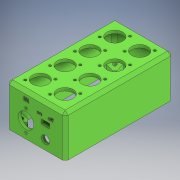
# Autodesk Inventor part: Case1
Saved by Autodesk Inventor 2020 (Build 240168000, 168)
## iProperties
Created: 2020-11-28
Part Number: Case1
Material: Generic
Document SubType Name: Modeling
Designer: Milosz
Density: 1 g/cm^3
Appearance: Default
Author: Milosz
## iProperties of the stored document _3DPrint.ipt
Created: 2020-11-29
Part Number: _3DPrint
Material: Generic
Document SubType Name: Modeling
Designer: Milosz
Density: 1 g/cm^3
Appearance: Default
Author: Milosz
Autodesk Inventor part; units mm, degrees
ref_plane "YZ Plane" through (0, 0, 0) normal (1, 0, 0) x (0, 1, 0)
ref_plane "XZ Plane" through (0, 0, 0) normal (0, 1, 0) x (-1, 0, 0)
ref_plane "XY Plane" through (0, 0, 0) normal (0, 0, 1) x (1, 0, 0)
sketch "Sketch1" plane through (0, 0, 0) normal (0, 1, 0) x (-1, 0, 0)
  circle A0 centre (21.5, -16.9) radius 8
  circle A1 centre (14.2219, -24.8454) radius 1.25
  circle A2 centre (28.7781, -8.9546) radius 1.25
  arc A3 (11.0876, -24.5315) -> (14.8089, -27.9403) centre (14.2219, -24.8454) ccw construction
  arc A4 (31.9108, -9.2842) -> (28.1911, -5.8597) centre (28.7781, -8.9546) ccw construction
  line L0 (31.0995, -16.9941) -> (31.9108, -9.2842) construction
  line L1 (28.1911, -5.8597) -> (19.7111, -7.4682) construction
  line L2 (11.9478, -15.9432) -> (11.0876, -24.5315) construction
  line L3 (23.2889, -26.3318) -> (14.8089, -27.9403) construction
  arc A5 (19.7111, -7.4682) -> (11.9478, -15.9432) centre (21.5, -16.9) ccw construction
  arc A6 (23.2889, -26.3318) -> (31.0995, -16.9941) centre (21.5, -16.9) ccw construction
  line L4 (35.5, -91.9) -> (35.5, -105.9) construction
  line L5 (35.5, -105.9) -> (21.5, -105.9) construction
  line L6 (-3.5, -16.9) -> (-17.5, -16.9) construction
  line L7 (-17.5, -16.9) -> (-17.5, -2.9) construction
  line L8 (-17.5, -2.9) -> (-3.5, -2.9) construction
  line L9 (-3.5, -2.9) -> (-3.5, -16.9) construction
  line L10 (35.5, -105.9) -> (-17.5, -105.9)
  line L11 (-17.5, -105.9) -> (-17.5, -2.9)
  line L12 (-17.5, -2.9) -> (35.5, -2.9)
  line L13 (35.5, -2.9) -> (35.5, -105.9)
  line L14 (28.1911, -30.8597) -> (19.7111, -32.4682) construction
  line L15 (23.2889, -51.3318) -> (14.8089, -52.9403) construction
  circle A7 centre (14.2219, -49.8454) radius 1.25
  circle A8 centre (28.7781, -33.9546) radius 1.25
  line L16 (31.0995, -41.9941) -> (31.9108, -34.2842) construction
  line L17 (11.9478, -40.9432) -> (11.0876, -49.5315) construction
  arc A9 (19.7111, -32.4682) -> (11.9478, -40.9432) centre (21.5, -41.9) ccw construction
  circle A10 centre (21.5, -41.9) radius 8
  arc A11 (11.0876, -49.5315) -> (14.8089, -52.9403) centre (14.2219, -49.8454) ccw construction
  arc A12 (31.9108, -34.2842) -> (28.1911, -30.8597) centre (28.7781, -33.9546) ccw construction
  arc A13 (23.2889, -51.3318) -> (31.0995, -41.9941) centre (21.5, -41.9) ccw construction
  line L18 (28.1911, -55.8597) -> (19.7111, -57.4682) construction
  line L19 (23.2889, -76.3318) -> (14.8089, -77.9403) construction
  circle A14 centre (14.2219, -74.8454) radius 1.25
  circle A15 centre (28.7781, -58.9546) radius 1.25
  line L20 (31.0995, -66.9941) -> (31.9108, -59.2842) construction
  line L21 (11.9478, -65.9432) -> (11.0876, -74.5315) construction
  arc A16 (19.7111, -57.4682) -> (11.9478, -65.9432) centre (21.5, -66.9) ccw construction
  circle A17 centre (21.5, -66.9) radius 8
  arc A18 (11.0876, -74.5315) -> (14.8089, -77.9403) centre (14.2219, -74.8454) ccw construction
  arc A19 (31.9108, -59.2842) -> (28.1911, -55.8597) centre (28.7781, -58.9546) ccw construction
  arc A20 (23.2889, -76.3318) -> (31.0995, -66.9941) centre (21.5, -66.9) ccw construction
  line L22 (28.1911, -80.8597) -> (19.7111, -82.4682) construction
  line L23 (23.2889, -101.3318) -> (14.8089, -102.9403) construction
  circle A21 centre (14.2219, -99.8454) radius 1.25
  circle A22 centre (28.7781, -83.9546) radius 1.25
  line L24 (31.0995, -91.9941) -> (31.9108, -84.2842) construction
  line L25 (11.9478, -90.9432) -> (11.0876, -99.5315) construction
  arc A23 (19.7111, -82.4682) -> (11.9478, -90.9432) centre (21.5, -91.9) ccw construction
  circle A24 centre (21.5, -91.9) radius 8
  arc A25 (11.0876, -99.5315) -> (14.8089, -102.9403) centre (14.2219, -99.8454) ccw construction
  arc A26 (31.9108, -84.2842) -> (28.1911, -80.8597) centre (28.7781, -83.9546) ccw construction
  arc A27 (23.2889, -101.3318) -> (31.0995, -91.9941) centre (21.5, -91.9) ccw construction
  line L26 (3.1911, -5.8597) -> (-5.2889, -7.4682) construction
  line L27 (-1.7111, -26.3318) -> (-10.1911, -27.9403) construction
  circle A28 centre (-10.7781, -24.8454) radius 1.25
  circle A29 centre (3.7781, -8.9546) radius 1.25
  line L28 (6.0995, -16.9941) -> (6.9108, -9.2842) construction
  line L29 (-13.0522, -15.9432) -> (-13.9124, -24.5315) construction
  arc A30 (-5.2889, -7.4682) -> (-13.0522, -15.9432) centre (-3.5, -16.9) ccw construction
  circle A31 centre (-3.5, -16.9) radius 8
  arc A32 (-13.9124, -24.5315) -> (-10.1911, -27.9403) centre (-10.7781, -24.8454) ccw construction
  arc A33 (6.9108, -9.2842) -> (3.1911, -5.8597) centre (3.7781, -8.9546) ccw construction
  arc A34 (-1.7111, -26.3318) -> (6.0995, -16.9941) centre (-3.5, -16.9) ccw construction
  line L30 (3.1911, -30.8597) -> (-5.2889, -32.4682) construction
  line L31 (-1.7111, -51.3318) -> (-10.1911, -52.9403) construction
  circle A35 centre (-10.7781, -49.8454) radius 1.25
  circle A36 centre (3.7781, -33.9546) radius 1.25
  line L32 (6.0995, -41.9941) -> (6.9108, -34.2842) construction
  line L33 (-13.0522, -40.9432) -> (-13.9124, -49.5315) construction
  arc A37 (-5.2889, -32.4682) -> (-13.0522, -40.9432) centre (-3.5, -41.9) ccw construction
  circle A38 centre (-3.5, -41.9) radius 8
  arc A39 (-13.9124, -49.5315) -> (-10.1911, -52.9403) centre (-10.7781, -49.8454) ccw construction
  arc A40 (6.9108, -34.2842) -> (3.1911, -30.8597) centre (3.7781, -33.9546) ccw construction
  arc A41 (-1.7111, -51.3318) -> (6.0995, -41.9941) centre (-3.5, -41.9) ccw construction
  line L34 (3.1911, -55.8597) -> (-5.2889, -57.4682) construction
  line L35 (-1.7111, -76.3318) -> (-10.1911, -77.9403) construction
  circle A42 centre (-10.7781, -74.8454) radius 1.25
  circle A43 centre (3.7781, -58.9546) radius 1.25
  line L36 (6.0995, -66.9941) -> (6.9108, -59.2842) construction
  line L37 (-13.0522, -65.9432) -> (-13.9124, -74.5315) construction
  arc A44 (-5.2889, -57.4682) -> (-13.0522, -65.9432) centre (-3.5, -66.9) ccw construction
  circle A45 centre (-3.5, -66.9) radius 8
  arc A46 (-13.9124, -74.5315) -> (-10.1911, -77.9403) centre (-10.7781, -74.8454) ccw construction
  arc A47 (6.9108, -59.2842) -> (3.1911, -55.8597) centre (3.7781, -58.9546) ccw construction
  arc A48 (-1.7111, -76.3318) -> (6.0995, -66.9941) centre (-3.5, -66.9) ccw construction
  line L38 (3.1911, -80.8597) -> (-5.2889, -82.4682) construction
  line L39 (-1.7111, -101.3318) -> (-10.1911, -102.9403) construction
  circle A49 centre (-10.7781, -99.8454) radius 1.25
  circle A50 centre (3.7781, -83.9546) radius 1.25
  line L40 (6.0995, -91.9941) -> (6.9108, -84.2842) construction
  line L41 (-13.0522, -90.9432) -> (-13.9124, -99.5315) construction
  arc A51 (-5.2889, -82.4682) -> (-13.0522, -90.9432) centre (-3.5, -91.9) ccw construction
  circle A52 centre (-3.5, -91.9) radius 8
  arc A53 (-13.9124, -99.5315) -> (-10.1911, -102.9403) centre (-10.7781, -99.8454) ccw construction
  arc A54 (6.9108, -84.2842) -> (3.1911, -80.8597) centre (3.7781, -83.9546) ccw construction
  arc A55 (-1.7111, -101.3318) -> (6.0995, -91.9941) centre (-3.5, -91.9) ccw construction
  line L42 (28.7781, -8.9546) -> (14.2219, -24.8454) construction
  point P0 (0, 0)
  point P1 (21.5, -16.9)
  point P2 (21.5, -41.9)
  point P3 (21.5, -66.9)
  point P4 (21.5, -91.9)
  point P5 (-3.5, -41.9)
  point P6 (-3.5, -66.9)
  point P7 (-3.5, -91.9)
  dimension "d0" = 16
  dimension "d3" = 2.5
  dimension "d4" = 2.5
  dimension "d6" = 6.3
  dimension "d7" = 6.3
  dimension "d9" = 9.6
  dimension "d10" = 9.6
  dimension "d19" = 14
  dimension "d20" = 14
  dimension "d21" = 14
  dimension "d22" = 14
  dimension "d25" = 25
  dimension "d28" = 25
  dimension "d55" = 10.775
  dimension "d56" = 10.775
  constraints: 86 end point, 64 point on circle, 56 centre point, 24 coincident, 7 tangent, 4 parallel, 3 horizontal, 2 perpendicular, 1 midpoint, 1 vertical, 182 other
  measures "d0" diameter of A0
  measures "d3" diameter of A1
  measures "d4" diameter of A2
  measures "d6" diameter of A3
  measures "d7" diameter of A4
  measures "d9" radius of A6
  measures "d10" radius of A5
  measures "d19" distance of L4.end L5.end
  measures "d20" distance of L4.start L4.end
  measures "d21" distance of L7.end L8.end
  measures "d22" distance of L6.end L7.end
  measures "d25" distance of L2.start L17.start
  measures "d28" distance of L2.start L29.start
  measures "d55" distance of A0.centre A1.centre
  measures "d56" distance of A2.centre A0.centre
extrude "Extrusion1" add sketch "Sketch1" along normal blind 3
sketch "Sketch2" plane through (0, 0, 0) normal (0, -1, 0) x (1, 0, 0)
  line L0 (-35.5, -105.9) -> (-35.5, -2.9) projected
  line L1 (-35.5, -2.9) -> (17.5, -2.9) projected
  line L2 (-35.5, -2.9) -> (17.5, -2.9) projected
  line L3 (17.5, -2.9) -> (-35.5, -2.9)
  line L4 (-35.5, -2.9) -> (-35.5, 0.1)
  line L5 (-35.5, 0.1) -> (17.5, 0.1)
  line L6 (17.5, 0.1) -> (17.5, -2.9)
  line L7 (-35.5, 0.1) -> (-38.5, 0.1)
  line L8 (-38.5, 0.1) -> (-38.5, -105.9)
  line L9 (-38.5, -105.9) -> (-35.5, -105.9)
  line L10 (-35.5, -105.9) -> (-35.5, 0.1)
  line L11 (-38.5, -105.9) -> (17.5, -105.9)
  line L12 (17.5, -105.9) -> (17.5, -108.9)
  line L13 (17.5, -108.9) -> (-38.5, -108.9)
  line L14 (-38.5, -108.9) -> (-38.5, -105.9)
  line L15 (17.5, -108.9) -> (20.5, -108.9)
  line L16 (20.5, -108.9) -> (20.5, 0.1)
  line L17 (20.5, 0.1) -> (17.5, 0.1)
  line L18 (17.5, 0.1) -> (17.5, -108.9)
  point P0 (0, 0)
  point P1 (17.5, -2.9)
  dimension "d33" = 3
  dimension "d34" = 3
  dimension "d35" = 3
  dimension "d36" = 3
  constraints: 32 end point, 8 parallel, 4 horizontal, 4 perpendicular, 2 point on line
  measures "d33" distance of L3.end L4.end
  measures "d34" distance of L9.end L8.end
  measures "d35" distance of L11.end L12.end
  measures "d36" distance of L17.end L16.end
extrude "Extrusion2" add sketch "Sketch2" along normal blind 40 and the other way blind 3 contours L9 L8 L7 L4 L0 | L11 L12 L13 L14 L9 | L4 L5 L6 L1 | L18 L6 L17 L16 L15 L12
chamfer "Chamfer1" distance 3 angle 45 16 edges at (-9, 3, 0.1) (-38.5, 3, -54.4) (-9, 3, -108.9) (20.5, 3, -54.4) (20.5, -18.5, -108.9) (-38.5, -18.5, -108.9) (20.5, -18.5, 0.1) (-38.5, -18.5, 0.1) (-35.5, -20, -2.9) (17.5, -20, -2.9) (17.5, -20, -105.9) (-35.5, -20, -105.9) (-9, 0, -2.9) (-35.5, 0, -54.4) (-9, 0, -105.9) (17.5, 0, -54.4)
sketch "Sketch3" plane through (0, 0, 0) normal (0, -1, 0) x (1, 0, 0)
  circle A0 centre (3.5, -91.9) radius 8 projected
  circle A1 centre (-3.7781, -83.9546) radius 1.25 projected
  circle A2 centre (10.7781, -99.8454) radius 1.25 projected
  circle A3 centre (3.5, -66.9) radius 8 projected
  circle A4 centre (-3.7781, -58.9546) radius 1.25 projected
  circle A5 centre (10.7781, -74.8454) radius 1.25 projected
  circle A6 centre (3.5, -41.9) radius 8 projected
  circle A7 centre (-3.7781, -33.9546) radius 1.25 projected
  circle A8 centre (10.7781, -49.8454) radius 1.25 projected
  circle A9 centre (3.5, -16.9) radius 8 projected
  circle A10 centre (-3.7781, -8.9546) radius 1.25 projected
  circle A11 centre (10.7781, -24.8454) radius 1.25 projected
  circle A12 centre (-21.5, -91.9) radius 8 projected
  circle A13 centre (-28.7781, -83.9546) radius 1.25 projected
  circle A14 centre (-14.2219, -99.8454) radius 1.25 projected
  circle A15 centre (-21.5, -66.9) radius 8 projected
  circle A16 centre (-28.7781, -58.9546) radius 1.25 projected
  circle A17 centre (-14.2219, -74.8454) radius 1.25 projected
  circle A18 centre (-21.5, -41.9) radius 8 projected
  circle A19 centre (-28.7781, -33.9546) radius 1.25 projected
  circle A20 centre (-14.2219, -49.8454) radius 1.25 projected
  circle A21 centre (-28.7781, -8.9546) radius 1.25 projected
  circle A22 centre (-14.2219, -24.8454) radius 1.25 projected
  circle A23 centre (-21.5, -16.9) radius 8 projected
  line L0 (14.5, -102.9) -> (-32.5, -102.9) projected
  line L1 (14.5, -5.9) -> (14.5, -102.9) projected
  line L2 (-32.5, -5.9) -> (14.5, -5.9) projected
  line L3 (-32.5, -102.9) -> (-32.5, -5.9) projected
  line L4 (-14.2219, -24.8454) -> (-21.5, -16.9) construction
  line L5 (-14.7713, -22.3652) -> (-12.3487, -23.1295)
  line L6 (-12.3487, -23.1295) -> (-11.7993, -25.6098)
  line L7 (-11.7993, -25.6098) -> (-13.6725, -27.3257)
  line L8 (-13.6725, -27.3257) -> (-16.0951, -26.5613)
  line L9 (-16.0951, -26.5613) -> (-16.6445, -24.0811)
  line L10 (-16.6445, -24.0811) -> (-14.7713, -22.3652)
  circle A24 centre (-28.7781, -8.9546) radius 1.25 construction
  line L11 (-28.7781, -8.9546) -> (-21.5, -16.9) construction
  line L12 (-28.2287, -11.4348) -> (-30.6513, -10.6705)
  line L13 (-30.6513, -10.6705) -> (-31.2007, -8.1902)
  line L14 (-31.2007, -8.1902) -> (-29.3275, -6.4743)
  line L15 (-29.3275, -6.4743) -> (-26.9049, -7.2387)
  line L16 (-26.9049, -7.2387) -> (-26.3555, -9.7189)
  line L17 (-26.3555, -9.7189) -> (-28.2287, -11.4348)
  point P0 (0, 0)
  point P1 (-14.1712, -24.9007)
  point P2 (-15.7079, -23.2232)
  point P3 (-27.2921, -10.5768)
  dimension "d45" = 4.4
  dimension "d46" = 4.4
  constraints: 28 end point, 2 coincident, 2 midpoint, 2 point on line, 26 other
  measures "d45" distance between parallel lines of L7 L10
  measures "d46" distance between parallel lines of L16 L13
extrude "Extrusion3" cut sketch "Sketch3" against normal blind 1 contours L5 L6 L7 L8 L9 L10 | L12 L13 L14 L15 L16 L17
pattern_linear "Rectangular Pattern1" count 4 spacing 25 along (0, 0, -1) count 2 spacing 25 along (1, 0, 0) of "Extrusion3"
sketch "Sketch4" plane through (0, -40, 0) normal (0, -1, 0) x (1, 0, 0)
  line L0 (17.5, -5.9) -> (17.5, -102.9) projected
  line L1 (17.5, -5.9) -> (17.5, -102.9) projected
  line L2 (14.5, -105.9) -> (17.5, -102.9) projected
  line L3 (14.5, -105.9) -> (-32.5, -105.9) projected
  line L4 (-35.5, -102.9) -> (-32.5, -105.9) projected
  line L5 (-35.5, -102.9) -> (-35.5, -5.9) projected
  line L6 (-32.5, -2.9) -> (-35.5, -5.9) projected
  line L7 (-32.5, -2.9) -> (14.5, -2.9) projected
  line L8 (17.5, -5.9) -> (14.5, -2.9) projected
  line L9 (20.5, -105.9) -> (17.5, -108.9) projected
  line L10 (20.5, -105.9) -> (20.5, -2.9) projected
  line L11 (17.5, 0.1) -> (20.5, -2.9) projected
  line L12 (17.5, 0.1) -> (-35.5, 0.1) projected
  line L13 (-38.5, -2.9) -> (-35.5, 0.1) projected
  line L14 (-38.5, -2.9) -> (-38.5, -105.9) projected
  line L15 (-35.5, -108.9) -> (-38.5, -105.9) projected
  line L16 (-35.5, -108.9) -> (17.5, -108.9) projected
  circle A0 centre (-31.1, -7.3) radius 1.75
  line L17 (-35.5, -2.9) -> (-35.5, -105.9) projected
  line L18 (-35.5, -2.9) -> (-26.7, -2.9)
  line L19 (-26.7, -2.9) -> (-26.7, -11.7)
  line L20 (-26.7, -11.7) -> (-35.5, -11.7)
  line L21 (-35.5, -11.7) -> (-35.5, -2.9)
  point P0 (0, 0)
  dimension "d57" = 3.5
  dimension "d58" = 8.8
  dimension "d59" = 8.8
  dimension "d60" = 4.4
  dimension "d61" = 4.4
  constraints: 8 end point, 2 parallel, 1 centre point, 1 horizontal, 1 perpendicular
  measures "d57" diameter of A0
  measures "d58" distance of L19.end L20.end
  measures "d59" distance of L18.end L19.end
  measures "d60" distance from line of L7 A0.centre
  measures "d61" distance from line of L21 A0.centre
extrude "Extrusion4" add sketch "Sketch4" against normal blind 7.05 contours L19 L20 L5 L6 L7
chamfer "Chamfer2" distance 2 angle 45 1 edges at (-26.7, -36.475, -11.7)
draft "FaceDraft1" angle 30 pull direction (0.7071068, 0, -0.7071068) faces at (-27.6003, -32.95, -6.4937) fixed edges at (-27.7, -32.95, -10.7)
sketch "Sketch5" plane through (0, -40, 0) normal (0, -1, 0) x (1, 0, 0)
  line L0 (20.5, -105.9) -> (17.5, -108.9) projected
  line L1 (20.5, -105.9) -> (20.5, -2.9) projected
  line L2 (17.5, 0.1) -> (20.5, -2.9) projected
  line L3 (17.5, 0.1) -> (-35.5, 0.1) projected
  line L4 (-38.5, -2.9) -> (-35.5, 0.1) projected
  line L5 (-38.5, -2.9) -> (-38.5, -105.9) projected
  line L6 (-35.5, -108.9) -> (-38.5, -105.9) projected
  line L7 (-35.5, -108.9) -> (17.5, -108.9) projected
  line L8 (-26.7, -9.7) -> (-28.7, -11.7) projected
  line L9 (-26.7, -9.7) -> (-26.7, -2.9) projected
  line L10 (-26.7, -2.9) -> (14.5, -2.9) projected
  line L11 (17.5, -5.9) -> (14.5, -2.9) projected
  line L12 (17.5, -5.9) -> (17.5, -102.9) projected
  line L13 (14.5, -105.9) -> (17.5, -102.9) projected
  line L14 (14.5, -105.9) -> (-32.5, -105.9) projected
  line L15 (-35.5, -102.9) -> (-32.5, -105.9) projected
  line L16 (-35.5, -102.9) -> (-35.5, -11.7) projected
  line L17 (-35.5, -11.7) -> (-28.7, -11.7) projected
  circle A0 centre (-31.1, -7.3) radius 1.75 projected
  line L18 (18.95, -3.542) -> (18.95, -105.258)
  line L19 (18.95, -105.258) -> (16.858, -107.35)
  line L20 (16.858, -107.35) -> (-34.858, -107.35)
  line L21 (-34.858, -107.35) -> (-36.95, -105.258)
  line L22 (-36.95, -105.258) -> (-36.95, -3.542)
  line L23 (-36.95, -3.542) -> (-34.858, -1.45)
  line L24 (-34.858, -1.45) -> (16.858, -1.45)
  line L25 (16.858, -1.45) -> (18.95, -3.542)
  point P0 (0, 0)
  dimension "d68" = 1.55
  constraints: 16 end point, 7 other
  measures "d68" distance between parallel lines of L1 L18
extrude "Extrusion5" cut sketch "Sketch5" against normal blind 1 contours L0 L7 L6 L5 L4 L3 L2 L1
sketch "Sketch7" plane through (-26.7, -40, -9.7) normal (0.7071068, 0, -0.7071068) x (-0.7071068, 0, -0.7071068)
  circle A0 centre (1.4142, 13.6083) radius 1.75
  line L0 (3.1642, 0) -> (-0.3358, 0)
  line L1 (3.1642, 0) -> (-0.3358, 13.6083) construction
  circle A1 centre (1.4142, 13.6083) radius 1.75 construction
  line L2 (3.1642, 13.6083) -> (-0.3358, 0) construction
  line L3 (1.4142, 6.8042) -> (1.4142, 0) construction
  line L4 (3.1642, 0) -> (-0.3358, 0) construction
  line L5 (-1.5858, 5.2) -> (4.4142, 5.2)
  line L6 (4.4142, 5.2) -> (4.4142, 2.5)
  line L7 (4.4142, 2.5) -> (-1.5858, 2.5)
  line L8 (-1.5858, 2.5) -> (-1.5858, 5.2)
  line L9 (-1.5858, 5.2) -> (4.4142, 2.5) construction
  line L10 (4.4142, 5.2) -> (-1.5858, 2.5) construction
  line L11 (-0.0651, 0) -> (2.8935, 0) construction
  point P0 (-25.7387, 40)
  point P1 (1.4142, 3.4021)
  point P2 (1.4142, 3.85)
  dimension "d73" = 6
  dimension "d74" = 2.7
  dimension "d75" = 2.5
  constraints: 20 end point, 5 midpoint, 2 parallel, 2 point on circle, 1 centre point, 1 horizontal, 1 perpendicular, 1 point on line, 1 vertical
  measures "d73" distance of L6.end L7.end
  measures "d74" distance of L5.end L6.end
  measures "d75" distance between parallel lines of L11 L7
extrude "Extrusion6" cut sketch "Sketch7" against normal up to surface (8.9095 mm away) contours L5 L6 L7 L8
chamfer "Chamfer3" distance 1 distance2 3 1 edges at (-29.2893, -37.5, -4.868) measured on face at (-29.2893, -37, -4.868)
chamfer "Chamfer4" distance 3 distance2 1 1 edges at (-33.532, -37.5, -9.1107) measured on face at (-33.1784, -37.5, -8.7571)
sketch "Sketch8" plane through (0, -40, 0) normal (0, -1, 0) x (1, 0, 0)
  line L0 (-36.95, -3.542) -> (-36.95, -105.258) projected
  line L1 (-36.95, -105.258) -> (-34.858, -107.35) projected
  line L2 (-34.858, -107.35) -> (16.858, -107.35) projected
  line L3 (16.858, -107.35) -> (18.95, -105.258) projected
  line L4 (18.95, -105.258) -> (18.95, -3.542) projected
  line L5 (18.95, -3.542) -> (16.858, -1.45) projected
  line L6 (16.858, -1.45) -> (-34.858, -1.45) projected
  line L7 (-34.858, -1.45) -> (-36.95, -3.542) projected
  line L8 (-26.7, -9.7) -> (-28.7, -11.7) projected
  line L9 (-26.7, -9.7) -> (-26.7, -2.9) projected
  line L10 (-26.7, -2.9) -> (14.5, -2.9) projected
  line L11 (17.5, -5.9) -> (14.5, -2.9) projected
  line L12 (17.5, -5.9) -> (17.5, -102.9) projected
  line L13 (14.5, -105.9) -> (17.5, -102.9) projected
  line L14 (14.5, -105.9) -> (-32.5, -105.9) projected
  line L15 (-35.5, -102.9) -> (-32.5, -105.9) projected
  line L16 (-35.5, -102.9) -> (-35.5, -11.7) projected
  line L17 (-35.5, -11.7) -> (-28.7, -11.7) projected
  circle A0 centre (-31.1, -7.3) radius 1.75 projected
  line L18 (17.5, -102.9) -> (17.5, -5.9) projected
  line L19 (17.5, -54.4) -> (-35.5, -54.4)
  line L20 (-35.5, -2.9) -> (-35.5, -105.9) projected
  line L21 (14.5, -105.9) -> (-32.5, -105.9) projected
  line L22 (-9, -105.9) -> (-9, -2.9)
  line L23 (-26.7, -2.9) -> (14.5, -2.9) projected
  point P0 (0, 0)
  constraints: 4 end point, 3 midpoint, 1 perpendicular, 1 point on line
ref_plane "Work Plane1" through (17.5, -40, -54.4) normal (0, 0, 1) x (-1, 0, 0)
ref_plane "Work Plane2" through (-9, -40, -105.9) normal (1, 0, 0) x (0, 0, 1)
mirror "Mirror1" about plane through (17.5, -40, -54.4) normal (0, 0, 1) of "Extrusion4", "Chamfer2", "Extrusion6", "Chamfer4", "Chamfer3", "FaceDraft1"
mirror "Mirror2" about plane through (-9, -40, -105.9) normal (1, 0, 0) of "Extrusion6", "Chamfer3", "Chamfer4", "Extrusion4", "FaceDraft1", "Chamfer2", "Mirror1"
sketch "Sketch10" plane through (14.5, -3, -2.9) normal (0, 0, -1) x (-1, 0, 0)
  circle A0 centre (33.25, -19.75) radius 7.75
  line L0 (50, -24.8061) -> (50, 0) projected
  line L1 (47, 3) -> (0, 3) projected
  line L2 (33.25, -5.3373) -> (33.25, -31.7007) construction
  line L3 (-2.358, -37) -> (49.358, -37) construction
  circle A1 centre (33.25, -8.975) radius 1.25
  circle A2 centre (33.25, -30.525) radius 1.25
  line L4 (33.25, -19.75) -> (3.6624, -19.75) construction
  circle A3 centre (13.7076, -26.75) radius 4
  line L5 (13.7076, -26.75) -> (13.7076, -32.2603) construction
  line L6 (13.7076, -26.75) -> (13.7076, -6.8032) construction
  line L7 (9.4576, -10.5) -> (17.9576, -10.5)
  line L8 (17.9576, -10.5) -> (17.9576, -15)
  line L9 (17.9576, -15) -> (9.4576, -15)
  line L10 (9.4576, -15) -> (9.4576, -10.5)
  line L11 (9.4576, -10.5) -> (17.9576, -15) construction
  line L12 (17.9576, -10.5) -> (9.4576, -15) construction
  point P0 (14.5, 3)
  point P1 (13.7076, -12.75)
  dimension "d86" = 15.5
  dimension "d87" = 16.75
  dimension "d88" = 22.75
  dimension "d89" = 2.5
  dimension "d90" = 2.5
  dimension "d91" = 10.775
  dimension "d92" = 10.775
  dimension "d95" = 8
  dimension "d103" = 7
  dimension "d106" = 8.5
  dimension "d107" = 4.5
  dimension "d108" = 7
  constraints: 20 end point, 4 centre point, 3 point on line, 3 vertical, 2 horizontal, 2 midpoint, 2 parallel, 2 perpendicular
  measures "d86" diameter of A0
  measures "d87" distance from line of L0 L4.start
  measures "d88" distance from line of L1 L4.start
  measures "d89" diameter of A1
  measures "d90" diameter of A2
  measures "d91" distance of A2.centre L4.start
  measures "d92" distance of A1.centre L4.start
  measures "d95" diameter of A3
  measures "d103" distance from line of L5.start L4
  measures "d106" distance of L8.end L9.end
  measures "d107" distance of L7.end L8.end
  measures "d108" distance from line of point (13.708, -12.75) L4
extrude "Extrusion7" cut sketch "Sketch10" against normal up to surface (3 mm away) contours A0 | A1 | A2
extrude "Extrusion8" cut sketch "Sketch10" against normal up to surface (3 mm away) contours A3
sketch "Sketch11" plane through (14.5, -3, -2.9) normal (0, 0, -1) x (-1, 0, 0)
  circle A0 centre (13.7076, -26.75) radius 4 projected
  circle A1 centre (33.25, -30.525) radius 1.25 projected
  circle A2 centre (33.25, -19.75) radius 7.75 projected
  circle A3 centre (33.25, -8.975) radius 1.25 projected
  line L0 (50, -36) -> (-3, -36) projected
  line L1 (-3, 3) -> (-3, -36) projected
  line L2 (50, 3) -> (-3, 3) projected
  line L3 (50, -36) -> (50, 3) projected
  circle A4 centre (33.25, -8.975) radius 1.25 construction
  line L4 (33.25, -8.975) -> (33.25, -30.525) construction
  line L5 (31.9798, -11.175) -> (30.7097, -8.975)
  line L6 (30.7097, -8.975) -> (31.9798, -6.775)
  line L7 (31.9798, -6.775) -> (34.5202, -6.775)
  line L8 (34.5202, -6.775) -> (35.7903, -8.975)
  line L9 (35.7903, -8.975) -> (34.5202, -11.175)
  line L10 (34.5202, -11.175) -> (31.9798, -11.175)
  line L11 (34.5202, -28.325) -> (35.7903, -30.525)
  line L12 (35.7903, -30.525) -> (34.5202, -32.725)
  line L13 (34.5202, -32.725) -> (31.9798, -32.725)
  line L14 (31.9798, -32.725) -> (30.7097, -30.525)
  line L15 (30.7097, -30.525) -> (31.9798, -28.325)
  line L16 (31.9798, -28.325) -> (34.5202, -28.325)
  point P0 (14.5, 3)
  point P1 (33.25, -11.175)
  point P2 (33.25, -28.325)
  dimension "d98" = 4.4
  dimension "d99" = 4.4
  constraints: 26 end point, 2 coincident, 2 midpoint, 2 point on line, 1 vertical, 26 other
  measures "d98" distance between parallel lines of L13 L16
  measures "d99" distance between parallel lines of L8 L5
extrude "Extrusion9" cut sketch "Sketch11" against normal blind 1 contours L5 L6 L7 L8 L9 L10 | L11 L12 L13 L14 L15 L16
extrude "Extrusion10" cut sketch "Sketch10" against normal up to surface (3 mm away) contours L7 L8 L9 L10
sketch "Sketch12" plane through (14.5, -3, -2.9) normal (0, 0, -1) x (-1, 0, 0)
  point P0 (14.5, 3)
sketch "Sketch13" plane through (-35.5, 0, 0.1) normal (0, 0, 1) x (1, 0, 0)
  line L0 (13.9336, -2.4788) -> (19.5664, -2.4788) construction
  line L1 (19.5664, -2.4788) -> (19.5664, -8.7517) construction
  line L2 (19.5664, -8.7517) -> (13.9336, -8.7517) construction
  line L3 (13.9336, -8.7517) -> (13.9336, -2.4788) construction
  circle A0 centre (16.75, -22.75) radius 7.75 projected
  line L4 (16.75, -22.75) -> (16.75, -11.7933) construction
  line L5 (13.9336, -2.4788) -> (19.5664, -8.7517) construction
  line L6 (13.9336, -8.7517) -> (19.5664, -2.4788) construction
  line L7 (27.516, -8.5202) -> (33.1488, -8.5202) construction
  line L8 (33.1488, -8.5202) -> (33.1488, -14.7932) construction
  line L9 (33.1488, -14.7932) -> (27.516, -14.7932) construction
  line L10 (27.516, -14.7932) -> (27.516, -8.5202) construction
  line L11 (38.5374, -13.9018) -> (38.5374, -7.6289) construction
  line L12 (38.5374, -7.6289) -> (44.1702, -7.6289) construction
  line L13 (44.1702, -7.6289) -> (44.1702, -13.9018) construction
  line L14 (44.1702, -13.9018) -> (38.5374, -13.9018) construction
  line L15 (40.5424, -18) -> (32.0424, -18) projected
  line L16 (32.0424, -18) -> (32.0424, -13.5) projected
  line L17 (32.0424, -13.5) -> (40.5424, -13.5) projected
  line L18 (40.5424, -13.5) -> (40.5424, -18) projected
  circle A1 centre (36.2924, -29.75) radius 4 projected
  circle A2 centre (16.75, -33.525) radius 1.25 projected
  circle A3 centre (16.75, -22.75) radius 7.75 projected
  circle A4 centre (16.75, -11.975) radius 1.25 projected
  line L19 (0, -39) -> (53, -39) projected
  line L20 (53, 0) -> (53, -39) projected
  line L21 (0, 0) -> (53, 0) projected
  line L22 (0, -39) -> (0, 0) projected
  line L23 (40.5424, -18) -> (32.0424, -13.5) construction
  line L24 (40.5424, -18) -> (32.0424, -18) projected
  line L25 (32.0424, -18) -> (40.5424, -13.5) construction
  line L26 (36.2924, -15.75) -> (36.2924, -7.6059) construction
  spline S0 degree 2 poles (15.1806, -6.3698) (15.1806, -6.3999) (15.1393, -6.4487) (15.0491, -6.4788) (14.8951, -6.4975) (14.775, -6.4975) knots 0 0 0 1 2 3 4 4 4
  spline S1 degree 2 poles (14.775, -6.4975) (14.6585, -6.4975) (14.5008, -6.4788) (14.4106, -6.4487) (14.3693, -6.3999) (14.3693, -6.3698) knots 0 0 0 1 2 3 4 4 4
  line L27 (14.3693, -6.3698) -> (14.3693, -2.6065)
  spline S2 degree 2 poles (14.3693, -2.6065) (14.3693, -2.5764) (14.4106, -2.5276) (14.5045, -2.4975) (14.6585, -2.4788) (14.775, -2.4788) knots 0 0 0 1 2 3 4 4 4
  spline S3 degree 2 poles (14.775, -2.4788) (14.8951, -2.4788) (15.0491, -2.4975) (15.1393, -2.5276) (15.1806, -2.5764) (15.1806, -2.6065) knots 0 0 0 1 2 3 4 4 4
  line L28 (15.1806, -2.6065) -> (15.1806, -6.3698)
  spline S4 degree 2 poles (19.3308, -6.1971) (19.3308, -6.2684) (19.282, -6.3773) (19.1994, -6.4525) (19.0829, -6.4863) (19.0266, -6.4863) knots 0 0 0 1 2 3 4 4 4
  line L29 (19.0266, -6.4863) -> (18.6811, -6.4863)
  spline S5 degree 2 poles (18.6811, -6.4863) (18.5759, -6.4863) (18.4181, -6.4412) (18.2867, -6.3285) (18.1628, -6.1332) (18.0839, -5.983) knots 0 0 0 1 2 3 4 4 4
  line L30 (18.0839, -5.983) -> (17.0923, -4.1201)
  spline S6 degree 2 poles (17.0923, -4.1201) (17.0059, -3.9548) (16.8294, -3.568) (16.7581, -3.3877) knots 0 0 0 1 2 2 2
  line L31 (16.7581, -3.3877) -> (16.7505, -3.3877)
  spline S7 degree 2 poles (16.7505, -3.3877) (16.7656, -3.6093) (16.7768, -4.0487) (16.7768, -4.2816) knots 0 0 0 1 2 2 2
  line L32 (16.7768, -4.2816) -> (16.7768, -6.3661)
  spline S8 degree 2 poles (16.7768, -6.3661) (16.7768, -6.3961) (16.743, -6.445) (16.6604, -6.4788) (16.5177, -6.4975) (16.4088, -6.4975) knots 0 0 0 1 2 3 4 4 4
  spline S9 degree 2 poles (16.4088, -6.4975) (16.2998, -6.4975) (16.1571, -6.4788) (16.0782, -6.445) (16.0482, -6.3961) (16.0482, -6.3661) knots 0 0 0 1 2 3 4 4 4
  line L33 (16.0482, -6.3661) -> (16.0482, -2.7867)
  spline S10 degree 2 poles (16.0482, -2.7867) (16.0482, -2.6403) (16.2172, -2.4975) (16.3412, -2.4975) knots 0 0 0 1 2 2 2
  line L34 (16.3412, -2.4975) -> (16.7731, -2.4975)
  spline S11 degree 2 poles (16.7731, -2.4975) (16.8895, -2.4975) (17.051, -2.5388) (17.175, -2.629) (17.2876, -2.7942) (17.3477, -2.9144) knots 0 0 0 1 2 3 4 4 4
  line L35 (17.3477, -2.9144) -> (18.1214, -4.368)
  spline S12 degree 2 poles (18.1214, -4.368) (18.189, -4.5032) (18.3205, -4.7586) (18.4444, -5.014) (18.5609, -5.2581) (18.6172, -5.382) knots 0 0 0 1 2 3 4 4 4
  line L36 (18.6172, -5.382) -> (18.621, -5.382)
  spline S13 degree 2 poles (18.621, -5.382) (18.6097, -5.168) (18.6022, -4.6985) (18.6022, -4.4844) knots 0 0 0 1 2 2 2
  line L37 (18.6022, -4.4844) -> (18.6022, -2.614)
  spline S14 degree 2 poles (18.6022, -2.614) (18.6022, -2.5839) (18.6397, -2.5351) (18.7261, -2.4975) (18.8651, -2.4825) (18.9778, -2.4825) knots 0 0 0 1 2 3 4 4 4
  spline S15 degree 2 poles (18.9778, -2.4825) (19.0829, -2.4825) (19.2219, -2.4975) (19.3008, -2.5351) (19.3308, -2.5839) (19.3308, -2.614) knots 0 0 0 1 2 3 4 4 4
  line L38 (19.3308, -2.614) -> (19.3308, -6.1971)
  spline S16 degree 2 poles (29.9274, -9.6801) (29.9274, -9.9464) (29.7871, -10.3874) (29.5007, -10.7053) (29.0683, -10.88) (28.779, -10.88) knots 0 0 0 1 2 3 4 4 4
  spline S17 degree 2 poles (28.779, -10.88) (28.5012, -10.88) (28.0888, -10.7254) (27.8168, -10.4304) (27.685, -9.998) (27.685, -9.7202) knots 0 0 0 1 2 3 4 4 4
  spline S18 degree 2 poles (27.685, -9.7202) (27.685, -9.4538) (27.8282, -9.0099) (28.1146, -8.6949) (28.5442, -8.5202) (28.8334, -8.5202) knots 0 0 0 1 2 3 4 4 4
  spline S19 degree 2 poles (28.8334, -8.5202) (29.1141, -8.5202) (29.5265, -8.672) (29.7957, -8.967) (29.9274, -9.3994) (29.9274, -9.6801) knots 0 0 0 1 2 3 4 4 4
  spline S20 degree 2 poles (29.3203, -9.703) (29.3203, -9.5483) (29.2716, -9.2877) (29.1542, -9.0958) (28.9594, -8.987) (28.8105, -8.987) knots 0 0 0 1 2 3 4 4 4
  spline S21 degree 2 poles (28.8105, -8.987) (28.6788, -8.987) (28.4812, -9.0844) (28.3552, -9.2677) (28.2921, -9.5283) (28.2921, -9.6944) knots 0 0 0 1 2 3 4 4 4
  spline S22 degree 2 poles (28.2921, -9.6944) (28.2921, -9.849) (28.3437, -10.1096) (28.4583, -10.3015) (28.6559, -10.4075) (28.8019, -10.4075) knots 0 0 0 1 2 3 4 4 4
  spline S23 degree 2 poles (28.8019, -10.4075) (28.9365, -10.4075) (29.1313, -10.3101) (29.2601, -10.1297) (29.3203, -9.8691) (29.3203, -9.703) knots 0 0 0 1 2 3 4 4 4
  spline S24 degree 2 poles (32.3932, -10.7454) (32.3932, -10.7683) (32.3645, -10.8056) (32.2987, -10.8285) (32.1841, -10.8399) (32.0982, -10.8399) knots 0 0 0 1 2 3 4 4 4
  spline S25 degree 2 poles (32.0982, -10.8399) (32.0123, -10.8399) (31.8977, -10.8285) (31.8319, -10.8056) (31.8032, -10.7683) (31.8032, -10.7454) knots 0 0 0 1 2 3 4 4 4
  line L39 (31.8032, -10.7454) -> (31.8032, -9.5512)
  spline S26 degree 2 poles (31.8032, -9.5512) (31.8032, -9.3994) (31.7574, -9.2247) (31.6744, -9.1016) (31.5398, -9.0328) (31.451, -9.0328) knots 0 0 0 1 2 3 4 4 4
  spline S27 degree 2 poles (31.451, -9.0328) (31.3393, -9.0328) (31.1073, -9.1961) (30.9842, -9.3536) knots 0 0 0 1 2 2 2
  line L40 (30.9842, -9.3536) -> (30.9842, -10.7454)
  spline S28 degree 2 poles (30.9842, -10.7454) (30.9842, -10.7683) (30.9555, -10.8056) (30.8868, -10.8285) (30.7751, -10.8399) (30.6892, -10.8399) knots 0 0 0 1 2 3 4 4 4
  spline S29 degree 2 poles (30.6892, -10.8399) (30.6033, -10.8399) (30.4916, -10.8285) (30.4229, -10.8056) (30.3942, -10.7683) (30.3942, -10.7454) knots 0 0 0 1 2 3 4 4 4
  line L41 (30.3942, -10.7454) -> (30.3942, -8.6548)
  spline S30 degree 2 poles (30.3942, -8.6548) (30.3942, -8.6319) (30.4171, -8.5947) (30.4773, -8.5718) (30.5746, -8.5603) (30.6462, -8.5603) knots 0 0 0 1 2 3 4 4 4
  spline S31 degree 2 poles (30.6462, -8.5603) (30.7207, -8.5603) (30.8209, -8.5718) (30.8753, -8.5947) (30.8983, -8.6319) (30.8983, -8.6548) knots 0 0 0 1 2 3 4 4 4
  line L42 (30.8983, -8.6548) -> (30.8983, -8.8954)
  spline S32 degree 2 poles (30.8983, -8.8954) (31.0701, -8.7092) (31.4309, -8.5202) (31.6257, -8.5202) knots 0 0 0 1 2 2 2
  spline S33 degree 2 poles (31.6257, -8.5202) (31.8405, -8.5202) (32.1326, -8.6605) (32.313, -8.9011) (32.3932, -9.2276) (32.3932, -9.4538) knots 0 0 0 1 2 3 4 4 4
  line L43 (32.3932, -9.4538) -> (32.3932, -10.7454)
  spline S34 degree 2 poles (40.9488, -9.7682) (40.9488, -10.0345) (40.8085, -10.4755) (40.5221, -10.7934) (40.0896, -10.9681) (39.8004, -10.9681) knots 0 0 0 1 2 3 4 4 4
  spline S35 degree 2 poles (39.8004, -10.9681) (39.5226, -10.9681) (39.1102, -10.8135) (38.8381, -10.5185) (38.7064, -10.0861) (38.7064, -9.8083) knots 0 0 0 1 2 3 4 4 4
  spline S36 degree 2 poles (38.7064, -9.8083) (38.7064, -9.5419) (38.8496, -9.098) (39.136, -8.783) (39.5656, -8.6083) (39.8548, -8.6083) knots 0 0 0 1 2 3 4 4 4
  spline S37 degree 2 poles (39.8548, -8.6083) (40.1355, -8.6083) (40.5479, -8.7601) (40.8171, -9.0551) (40.9488, -9.4875) (40.9488, -9.7682) knots 0 0 0 1 2 3 4 4 4
  spline S38 degree 2 poles (40.3417, -9.7911) (40.3417, -9.6364) (40.293, -9.3758) (40.1756, -9.1839) (39.9808, -9.0751) (39.8319, -9.0751) knots 0 0 0 1 2 3 4 4 4
  spline S39 degree 2 poles (39.8319, -9.0751) (39.7002, -9.0751) (39.5026, -9.1725) (39.3765, -9.3558) (39.3135, -9.6164) (39.3135, -9.7825) knots 0 0 0 1 2 3 4 4 4
  spline S40 degree 2 poles (39.3135, -9.7825) (39.3135, -9.9371) (39.3651, -10.1977) (39.4796, -10.3896) (39.6773, -10.4956) (39.8233, -10.4956) knots 0 0 0 1 2 3 4 4 4
  spline S41 degree 2 poles (39.8233, -10.4956) (39.9579, -10.4956) (40.1527, -10.3982) (40.2815, -10.2178) (40.3417, -9.9572) (40.3417, -9.7911) knots 0 0 0 1 2 3 4 4 4
  spline S42 degree 2 poles (42.6786, -7.9439) (42.6786, -8.0126) (42.67, -8.0957) (42.6499, -8.1386) (42.627, -8.1558) (42.6127, -8.1558) knots 0 0 0 1 2 3 4 4 4
  spline S43 degree 2 poles (42.6127, -8.1558) (42.5955, -8.1558) (42.5554, -8.1386) (42.4981, -8.1214) (42.418, -8.1043) (42.3635, -8.1043) knots 0 0 0 1 2 3 4 4 4
  spline S44 degree 2 poles (42.3635, -8.1043) (42.3005, -8.1043) (42.2089, -8.1444) (42.1488, -8.2303) (42.1201, -8.3677) (42.1201, -8.468) knots 0 0 0 1 2 3 4 4 4
  line L44 (42.1201, -8.468) -> (42.1201, -8.6599)
  line L45 (42.1201, -8.6599) -> (42.5039, -8.6599)
  spline S45 degree 2 poles (42.5039, -8.6599) (42.5239, -8.6599) (42.5612, -8.6828) (42.5841, -8.7372) (42.5955, -8.8317) (42.5955, -8.8976) knots 0 0 0 1 2 3 4 4 4
  spline S46 degree 2 poles (42.5955, -8.8976) (42.5955, -9.0293) (42.5497, -9.1381) (42.5039, -9.1381) knots 0 0 0 1 2 2 2
  line L46 (42.5039, -9.1381) -> (42.1201, -9.1381)
  line L47 (42.1201, -9.1381) -> (42.1201, -10.8335)
  spline S47 degree 2 poles (42.1201, -10.8335) (42.1201, -10.8564) (42.0915, -10.8937) (42.0256, -10.9166) (41.9082, -10.928) (41.8251, -10.928) knots 0 0 0 1 2 3 4 4 4
  spline S48 degree 2 poles (41.8251, -10.928) (41.7392, -10.928) (41.6247, -10.9166) (41.5559, -10.8937) (41.5302, -10.8564) (41.5302, -10.8335) knots 0 0 0 1 2 3 4 4 4
  line L48 (41.5302, -10.8335) -> (41.5302, -9.1381)
  line L49 (41.5302, -9.1381) -> (41.2667, -9.1381)
  spline S49 degree 2 poles (41.2667, -9.1381) (41.2237, -9.1381) (41.1779, -9.0293) (41.1779, -8.8976) knots 0 0 0 1 2 2 2
  spline S50 degree 2 poles (41.1779, -8.8976) (41.1779, -8.8317) (41.1894, -8.7372) (41.2094, -8.6828) (41.2466, -8.6599) (41.2696, -8.6599) knots 0 0 0 1 2 3 4 4 4
  line L50 (41.2696, -8.6599) -> (41.5302, -8.6599)
  line L51 (41.5302, -8.6599) -> (41.5302, -8.4852)
  spline S51 degree 2 poles (41.5302, -8.4852) (41.5302, -8.2704) (41.6161, -7.9496) (41.7965, -7.7377) (42.0743, -7.6289) (42.2662, -7.6289) knots 0 0 0 1 2 3 4 4 4
  spline S52 degree 2 poles (42.2662, -7.6289) (42.3578, -7.6289) (42.5211, -7.6604) (42.6156, -7.6947) (42.6471, -7.7262) (42.67, -7.7835) (42.6786, -7.8752) (42.6786, -7.9439) knots 0 0 0 1 2 3 4 5 6 6 6
  spline S53 degree 2 poles (44.1993, -7.9439) (44.1993, -8.0126) (44.1907, -8.0957) (44.1706, -8.1386) (44.1477, -8.1558) (44.1334, -8.1558) knots 0 0 0 1 2 3 4 4 4
  spline S54 degree 2 poles (44.1334, -8.1558) (44.1162, -8.1558) (44.0761, -8.1386) (44.0189, -8.1214) (43.9387, -8.1043) (43.8842, -8.1043) knots 0 0 0 1 2 3 4 4 4
  spline S55 degree 2 poles (43.8842, -8.1043) (43.8212, -8.1043) (43.7296, -8.1444) (43.6695, -8.2303) (43.6408, -8.3677) (43.6408, -8.468) knots 0 0 0 1 2 3 4 4 4
  line L52 (43.6408, -8.468) -> (43.6408, -8.6599)
  line L53 (43.6408, -8.6599) -> (44.0246, -8.6599)
  spline S56 degree 2 poles (44.0246, -8.6599) (44.0446, -8.6599) (44.0819, -8.6828) (44.1048, -8.7372) (44.1162, -8.8317) (44.1162, -8.8976) knots 0 0 0 1 2 3 4 4 4
  spline S57 degree 2 poles (44.1162, -8.8976) (44.1162, -9.0293) (44.0704, -9.1381) (44.0246, -9.1381) knots 0 0 0 1 2 2 2
  line L54 (44.0246, -9.1381) -> (43.6408, -9.1381)
  line L55 (43.6408, -9.1381) -> (43.6408, -10.8335)
  spline S58 degree 2 poles (43.6408, -10.8335) (43.6408, -10.8564) (43.6122, -10.8937) (43.5463, -10.9166) (43.4289, -10.928) (43.3458, -10.928) knots 0 0 0 1 2 3 4 4 4
  spline S59 degree 2 poles (43.3458, -10.928) (43.2599, -10.928) (43.1454, -10.9166) (43.0766, -10.8937) (43.0509, -10.8564) (43.0509, -10.8335) knots 0 0 0 1 2 3 4 4 4
  line L56 (43.0509, -10.8335) -> (43.0509, -9.1381)
  line L57 (43.0509, -9.1381) -> (42.7874, -9.1381)
  spline S60 degree 2 poles (42.7874, -9.1381) (42.7444, -9.1381) (42.6986, -9.0293) (42.6986, -8.8976) knots 0 0 0 1 2 2 2
  spline S61 degree 2 poles (42.6986, -8.8976) (42.6986, -8.8317) (42.7101, -8.7372) (42.7301, -8.6828) (42.7673, -8.6599) (42.7903, -8.6599) knots 0 0 0 1 2 3 4 4 4
  line L58 (42.7903, -8.6599) -> (43.0509, -8.6599)
  line L59 (43.0509, -8.6599) -> (43.0509, -8.4852)
  spline S62 degree 2 poles (43.0509, -8.4852) (43.0509, -8.2704) (43.1368, -7.9496) (43.3172, -7.7377) (43.595, -7.6289) (43.7869, -7.6289) knots 0 0 0 1 2 3 4 4 4
  spline S63 degree 2 poles (43.7869, -7.6289) (43.8785, -7.6289) (44.0418, -7.6604) (44.1363, -7.6947) (44.1678, -7.7262) (44.1907, -7.7835) (44.1993, -7.8752) (44.1993, -7.9439) knots 0 0 0 1 2 3 4 5 6 6 6
  point P0 (35.5, 0)
  point P1 (16.75, -5.6152)
  dimension "d111" = 5.6327
  dimension "d112" = 5.6327
  dimension "d113" = 5.6327
  constraints: 12 end point, 2 midpoint, 2 vertical, 1 point on line, 6 other
  measures "d111" distance of L0.start L0.end
  measures "d112" distance of L10.end L7.end
  measures "d113" distance of L11.end L12.end
extrude "Extrusion11" cut sketch "Sketch13" against normal blind 0.4 contours S0 S1 L27 S2 S3 L28 | S4 L29 S5 L30 S6 L31 S7 L32 S8 S9 L33 S10 L34 S11 L35 S12 L36 S13 L37 S14 S15 L38 | S16 S17 S18 S19 | S24 S25 L39 S26 S27 L40 S28 S29 L41 S30 S31 L42 S32 S33 L43 | S34 S35 S36 S37 | S42 S43 S44 L44 L45 S45 S46 L46 L47 S47 S48 L48 L49 S49 S50 L50 L51 S51 S52 | S53 S54 S55 L52 L53 S56 S57 L54 L55 S58 S59 L56 L57 S60 S61 L58 L59 S62 S63
sketch "Sketch14" plane through (14.5, -3, -2.9) normal (0, 0, -1) x (-1, 0, 0)
  line L0 (7.8799, -5.468) -> (7.8799, -5.6599) projected
  line L1 (7.8799, -5.6599) -> (7.4961, -5.6599) projected
  line L2 (7.4961, -6.1381) -> (7.8799, -6.1381) projected
  line L3 (7.8799, -6.1381) -> (7.8799, -7.8335) projected
  line L4 (8.4698, -7.8335) -> (8.4698, -6.1381) projected
  line L5 (8.4698, -6.1381) -> (8.7333, -6.1381) projected
  line L6 (8.7304, -5.6599) -> (8.4698, -5.6599) projected
  line L7 (8.4698, -5.6599) -> (8.4698, -5.4852) projected
  line L8 (30.6692, 0.386) -> (30.6692, -3.1971) projected
  line L9 (30.9734, -3.4863) -> (31.3189, -3.4863) projected
  line L10 (31.9161, -2.983) -> (32.9077, -1.1201) projected
  line L11 (33.2419, -0.3877) -> (33.2495, -0.3877) projected
  line L12 (33.2232, -1.2816) -> (33.2232, -3.3661) projected
  line L13 (33.9518, -3.3661) -> (33.9518, 0.2133) projected
  line L14 (33.6588, 0.5025) -> (33.2269, 0.5025) projected
  line L15 (32.6523, 0.0856) -> (31.8786, -1.368) projected
  line L16 (31.3828, -2.382) -> (31.379, -2.382) projected
  line L17 (31.3978, -1.4844) -> (31.3978, 0.386) projected
  line L18 (34.8194, 0.3935) -> (34.8194, -3.3698) projected
  line L19 (35.6307, -3.3698) -> (35.6307, 0.3935) projected
  line L20 (16.6924, -7.7454) -> (16.6924, -7.8399) projected
  line L21 (17.9018, -7.893) -> (18.1968, -7.893) projected
  line L22 (18.1968, -7.7454) -> (18.1968, -6.5512) projected
  line L23 (18.1284, -7.7454) -> (18.1284, -7.8399) projected
  line L24 (19.3108, -7.893) -> (19.6058, -7.893) projected
  line L25 (18.8452, -5.5603) -> (18.8452, -5.6548) projected
  line L26 (19.1017, -5.6548) -> (19.1017, -5.8954) projected
  line L27 (18.1284, -5.8954) -> (18.1284, -5.5202) projected
  line L28 (6.3592, -5.468) -> (6.3592, -5.6599) projected
  line L29 (6.3592, -5.6599) -> (5.9754, -5.6599) projected
  line L30 (5.9754, -6.1381) -> (6.3592, -6.1381) projected
  line L31 (6.3592, -6.1381) -> (6.3592, -7.8335) projected
  line L32 (6.9491, -7.8335) -> (6.9491, -6.1381) projected
  line L33 (6.9491, -6.1381) -> (7.2126, -6.1381) projected
  line L34 (7.2097, -5.6599) -> (6.9491, -5.6599) projected
  line L35 (6.9491, -5.6599) -> (6.9491, -5.4852) projected
  line L36 (9.4576, -15) -> (17.9576, -15) projected
  line L37 (17.9576, -15) -> (17.9576, -10.5) projected
  line L38 (17.9576, -10.5) -> (9.4576, -10.5) projected
  line L39 (9.4576, -10.5) -> (9.4576, -15) projected
  circle A0 centre (13.7076, -26.75) radius 4 projected
  circle A1 centre (33.25, -30.525) radius 1.25 projected
  circle A2 centre (33.25, -19.75) radius 7.75 projected
  circle A3 centre (33.25, -8.975) radius 1.25 projected
  line L40 (50, -36) -> (-3, -36) projected
  line L41 (-3, 3) -> (-3, -36) projected
  line L42 (50, 3) -> (-3, 3) projected
  line L43 (50, -36) -> (50, 3) projected
  line L44 (9.4576, -10.5) -> (9.4576, -15) construction
  line L45 (17.9576, -15) -> (17.9576, -10.5) construction
  line L46 (9.4576, -15) -> (17.9576, -10.5) construction
  line L47 (17.9576, -10.5) -> (9.4576, -10.5) construction
  line L48 (17.9576, -10.5) -> (9.4576, -10.5) construction
  line L49 (9.4576, -10.5) -> (17.9576, -15) construction
  line L50 (21.9576, -16.75) -> (5.4576, -16.75)
  line L51 (5.4576, -16.75) -> (5.4576, -8.75)
  line L52 (5.4576, -8.75) -> (21.9576, -8.75)
  line L53 (21.9576, -8.75) -> (21.9576, -16.75)
  line L54 (21.9576, -16.75) -> (5.4576, -8.75) construction
  line L55 (5.4576, -16.75) -> (21.9576, -8.75) construction
  line L56 (23.9576, -6.75) -> (3.4576, -6.75)
  line L57 (3.4576, -6.75) -> (3.4576, -18.75)
  line L58 (3.4576, -18.75) -> (23.9576, -18.75)
  line L59 (23.9576, -18.75) -> (23.9576, -6.75)
  line L60 (19.6058, -7.7454) -> (19.6058, -5.6548) projected
  point P0 (14.5, 3)
  point P1 (17.9018, -7.8399)
  point P2 (19.3108, -7.8399)
  point P3 (13.7076, -12.75)
  dimension "d114" = 16.5
  dimension "d115" = 8
  dimension "d116" = 2
  constraints: 26 end point, 5 equal length, 3 midpoint, 2 perpendicular, 2 vertical alignment, 1 horizontal, 53 other
  measures "d114" distance of L50.start L50.end
  measures "d115" distance of L50.end L51.end
  measures "d116" distance between parallel lines of L52 L56
extrude "Extrusion12" add sketch "Sketch14" along normal blind 4 contours L59 L58 L57 L56
draft "FaceDraft3" angle 30 pull direction (0, 0, -1) faces at (-2.6243, -9.75, -5.5667) fixed edges at (0.7924, -9.75, -6.9)
equation "\"d4\" = d3"
equation "\"d56\" = d55"
equation "\"d59\" = d58"
equation "\"d60\" = 0.5 * d59"
equation "\"d61\" = 0.5 * d59"
body "Solid1"
